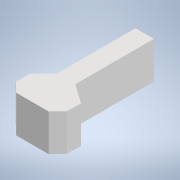
# Autodesk Inventor part: ДИ 00.00.06
Saved by Autodesk Inventor 2021.2 (Build 252289000, 289)
## iProperties
Created: 2021-10-12
Part Number: ДИ 00.00.06
Material: Типовые
Document SubType Name: Modeling
Designer: Surflay
Density: 1 g/cm^3
Appearance: По умолчанию
Author: Surflay
Autodesk Inventor part; units mm, degrees
ref_plane "YZ Plane" through (0, 0, 0) normal (1, 0, 0) x (0, 1, 0)
ref_plane "XZ Plane" through (0, 0, 0) normal (0, 1, 0) x (-1, 0, 0)
ref_plane "XY Plane" through (0, 0, 0) normal (0, 0, 1) x (1, 0, 0)
sketch "Эскиз1" plane through (0, 0, 0) normal (0, 0, 1) x (1, 0, 0)
  arc A0 (113.5, 24) -> (93.5, 4) centre (113.5, 4) ccw projected
  arc A1 (93.5, -1) -> (113.5, -21) centre (113.5, -1) ccw projected
  line L0 (93.5, 4) -> (93.5, -1) projected
  line L1 (88.5, 11.5) -> (28.5, 11.5)
  line L2 (28.5, 11.5) -> (28.5, -8.5)
  line L3 (28.5, -8.5) -> (88.5, -8.5)
  line L4 (88.5, -8.5) -> (88.5, 11.5)
  line L5 (-123.5, 102) -> (-123.5, -102) projected
  line L6 (-123.5, -102) -> (123.5, -102) projected
  line L7 (123.5, -102) -> (123.5, -100.4305) projected
  line L8 (123.5, -100.4305) -> (123.5, 102) projected
  line L9 (123.5, 102) -> (-123.5, 102) projected
  point P0 (0, 0)
  point P1 (88.5, 1.5)
  point P2 (93.5, 1.5)
  dimension "d0" = 20
  dimension "d1" = 60
  dimension "d2" = 5
  constraints: 8 end point, 2 midpoint, 2 parallel, 1 horizontal, 1 horizontal alignment, 1 perpendicular
  measures "d0" distance between parallel lines of L3 L1
  measures "d1" distance between parallel lines of L2 L4
  measures "d2" distance between parallel lines of L4 L0
extrude "Выдавливание1" add sketch "Эскиз1" along normal blind 30 contours L4 L3 L2 L1
sketch "Эскиз2" plane through (28.5, -8.5, 0) normal (0, -1, 0) x (1, 0, 0)
  line L0 (0, 0) -> (60, 0) projected
  line L1 (60, 0) -> (60, 3.0763)
  line L2 (60, 3.0763) -> (60, 10)
  line L3 (60, 10) -> (40, 20)
  line L4 (40, 20) -> (40, 25)
  line L5 (40, 25) -> (15, 25)
  line L6 (15, 25) -> (15, 20)
  line L7 (15, 20) -> (5, 10)
  line L8 (5, 10) -> (5, 0)
  line L9 (60, 0) -> (60, 30) projected
  point P0 (-28.5, 0)
  dimension "d6" = 25
  dimension "d7" = 5
  dimension "d8" = 5
  dimension "d9" = 20
  dimension "d10" = 10
  dimension "d11" = 10
  dimension "d12" = 10
  dimension "d13" = 25
  constraints: 16 end point, 3 perpendicular, 2 parallel, 2 point on line
  measures "d6" distance of L4.end L5.end
  measures "d7" distance of L5.end L6.end
  measures "d8" distance of L3.end L4.end
  measures "d9" horizontal distance of L2.end L3.end
  measures "d10" horizontal distance of L6.end L7.end
  measures "d11" horizontal distance of L6.end L7.end
  measures "d12" vertical distance of L2.end L3.end
  measures "d13" distance between parallel lines of L0 L5
extrude "Выдавливание2" cut sketch "Эскиз2" against normal blind 30 keep common part
sketch "Эскиз3" plane through (43.5, -8.5, 25) normal (0, 0, 1) x (1, 0, 0)
  line L0 (5, 14) -> (20, 14)
  line L1 (20, 14) -> (20, 6)
  line L2 (20, 6) -> (5, 6)
  line L3 (5, 6) -> (5, 14)
  line L4 (25, 20) -> (0, 20) projected
  line L5 (0, 0) -> (0, 20) projected
  point P0 (-43.5, 8.5)
  dimension "d16" = 8
  dimension "d17" = 15
  dimension "d18" = 6
  dimension "d19" = 25
  dimension "d20" = 20
  dimension "d21" = 5
  constraints: 8 end point, 2 parallel, 1 horizontal, 1 perpendicular
  measures "d16" distance between parallel lines of L2 L0
  measures "d17" distance between parallel lines of L1 L3
  measures "d18" distance between parallel lines of L4 L0
  measures "d19" distance of L4.start L4.end
  measures "d20" distance of L5.start L4.end
  measures "d21" distance between parallel lines of L5 L3
extrude "Выдавливание3" add sketch "Эскиз3" along normal blind 25
sketch "Эскиз4" plane through (48.5, -2.5, 25) normal (0, -1, 0) x (1, 0, 0)
  line L0 (15, 0) -> (0, 0) projected
  line L1 (5.5312, 0) -> (5.5312, 17)
  line L2 (5.5312, 17) -> (2.6422, 20)
  line L3 (2.6422, 20) -> (2.6422, 23)
  line L4 (2.6422, 23) -> (4.719, 25)
  line L5 (4.719, 25) -> (11.719, 25)
  line L6 (0, 25) -> (15, 25) projected
  line L7 (11.719, 25) -> (13.645, 23)
  line L8 (13.645, 23) -> (13.7498, 20)
  line L9 (13.7498, 20) -> (9.5312, 17)
  line L10 (9.5312, 17) -> (9.5312, 0)
  line L11 (-5, 0) -> (20, 0) projected
  line L12 (0, 0) -> (0, 25) projected
  line L13 (5.5312, 0) -> (9.5312, 0)
  line L14 (20, -5) -> (40, -15) projected
  line L15 (20, 0) -> (20, -5) projected
  line L16 (-5, 0) -> (20, 0) projected
  line L17 (-5, -5) -> (-5, 0) projected
  line L18 (-15, -15) -> (-5, -5) projected
  line L19 (-15, -25) -> (-15, -15) projected
  line L20 (-15, -25) -> (40, -25) projected
  line L21 (40, -25) -> (40, -15) projected
  point P0 (-48.5, -25)
  point P1 (9.5312, 0)
  dimension "d24" = 2
  dimension "d25" = 7
  dimension "d26" = 17
  dimension "d27" = 17
  dimension "d28" = 3
  dimension "d29" = 3
  dimension "d30" = 3
  dimension "d31" = 3
  dimension "d32" = 2
  dimension "d33" = 4
  dimension "d34" = 11.1076
  dimension "d35" = 2.6422
  constraints: 20 end point, 3 point on line, 2 collinear, 2 parallel, 2 perpendicular, 1 vertical
  measures "d24" angle of L3 L8
  measures "d25" distance of L4.end L5.end
  measures "d26" distance of L9.end L10.end
  measures "d27" distance of L1.start L1.end
  measures "d28" vertical distance of L8.end L9.end
  measures "d29" vertical distance of L1.end L2.end
  measures "d30" distance of L2.end L3.end
  measures "d31" vertical distance of L7.end L8.end
  measures "d32" vertical distance of L5.end L7.end
  measures "d33" distance between parallel lines of L1 L10
  measures "d34" distance of L2.end L8.end
  measures "d35" distance between parallel lines of L12 L3
extrude "Выдавливание4" cut sketch "Эскиз4" against normal through all both and the other way through all contours L11 L15 L14 L21 L20 L19 L18 L17 L0 | L0 L1 L2 L3 L4 L5 L7 L8 L9 L10 keep common part
equation "\"d18\" = -0.5 * d16 + 0.5 * d20"
equation "\"d21\" = -0.5 * d17 + 0.5 * d19"
